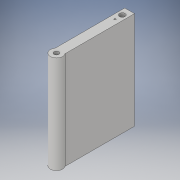
# Autodesk Inventor part: Gripper
Saved by Autodesk Inventor 2019 (Build 230136000, 136)
## iProperties
Created: 2019-09-29
Part Number: Gripper
Material: Generic
Document SubType Name: Modeling
Designer: james
Density: 1 g/cm^3
Appearance: Default
Author: james
Autodesk Inventor part; units mm, degrees
ref_plane "YZ Plane" through (0, 0, 0) normal (1, 0, 0) x (0, 1, 0)
ref_plane "XZ Plane" through (0, 0, 0) normal (0, 1, 0) x (-1, 0, 0)
ref_plane "XY Plane" through (0, 0, 0) normal (0, 0, 1) x (1, 0, 0)
sketch "Sketch1" plane through (0, 0, 0) normal (0, 1, 0) x (-1, 0, 0)
  circle A0 centre (17.2567, 94.6354) radius 6.35
  line L0 (22.3367, 94.6354) -> (12.1767, 94.6354)
  line L1 (12.1767, 94.6354) -> (12.1767, 18.4354)
  line L2 (12.1767, 18.4354) -> (22.3367, 18.4354)
  line L3 (22.3367, 18.4354) -> (22.3367, 94.6354)
  point P0 (0, 0)
  dimension "d0" = 12.7
  dimension "d1" = 76.2
  dimension "d2" = 0
  dimension "d3" = 10.16
  dimension "d4" = 5.08
  constraints: 8 end point, 2 parallel, 1 centre point, 1 horizontal, 1 perpendicular
  measures "d0" diameter of A0
  measures "d1" distance of L2.end L0.start
  measures "d2" distance from line of A0.centre L0
  measures "d3" distance of L1.end L2.end
  measures "d4" distance from line of L3 A0.centre
extrude "Extrusion1" add sketch "Sketch1" along normal blind 101.6
sketch "Sketch2" plane through (0, 101.6, 0) normal (0, 1, 0) x (1, 0, 0)
  arc A0 (-22.3367, -90.8254) -> (-12.1767, -90.8254) centre (-17.2567, -94.6354) ccw projected
  circle A1 centre (-17.2567, -94.6354) radius 2.54
  point P0 (0, 0)
  dimension "d7" = 5.08
  constraints: 1 centre point, 1 coincident
  measures "d7" diameter of A1
extrude "Extrusion2" cut sketch "Sketch2" against normal blind 482.6
sketch "Sketch3" plane through (0, 101.6, 0) normal (0, 1, 0) x (1, 0, 0)
  circle A0 centre (-17.2567, -26.0554) radius 2.8969
  line L0 (-12.1767, -18.4354) -> (-22.3367, -18.4354) projected
  line L1 (-22.3367, -18.4354) -> (-22.3367, -90.8254) projected
  point P0 (0, 0)
  dimension "d10" = 7.62
  dimension "d11" = 5.08
  constraints: 1 centre point
  measures "d10" distance from line of L0 A0.centre
  measures "d11" distance from line of L1 A0.centre
extrude "Extrusion3" cut sketch "Sketch3" against normal blind 482.6
sketch "Sketch4" plane through (0, 101.6, 0) normal (0, 1, 0) x (1, 0, 0)
  circle A0 centre (-17.2567, -33.6754) radius 2.6633
  line L0 (-12.1767, -90.8254) -> (-12.1767, -18.4354) projected
  line L1 (-12.1767, -18.4354) -> (-22.3367, -18.4354) projected
  point P0 (0, 0)
  dimension "d14" = 5.08
  dimension "d15" = 15.24
  constraints: 1 centre point, 1 coincident
  measures "d14" distance from line of L0 A0.centre
  measures "d15" distance from line of L1 point (-17.257, -33.675)
hole "Hole1" at (-17.2567, 101.6, 33.6754) direction (0, -1, 0) diameter 1.778 end through all
body "Solid1"
